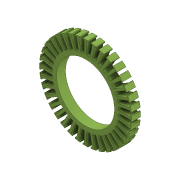
# Autodesk Inventor part: stator
Saved by Autodesk Inventor 2020 (Build 240168000, 168)
## iProperties
Created: 2020-05-19
Part Number: stator
Material: Generic
Document SubType Name: Modeling
Designer: Kostic
Density: 1 g/cm^3
Appearance: Olive Green
Author: Kostic
Autodesk Inventor part; units mm, degrees
ref_plane "YZ Plane" through (0, 0, 0) normal (1, 0, 0) x (0, 1, 0)
ref_plane "XZ Plane" through (0, 0, 0) normal (0, 1, 0) x (-1, 0, 0)
ref_plane "XY Plane" through (0, 0, 0) normal (0, 0, 1) x (1, 0, 0)
sketch "Sketch1" plane through (0, 0, 0) normal (0, 0, 1) x (1, 0, 0)
  circle A0 centre (0, 0) radius 26
  circle A1 centre (0, 0) radius 30
  line L0 (-1.1, 29.9798) -> (1.1, 29.9798)
  line L1 (1.1, 29.9798) -> (1.1, 41.4854)
  line L2 (1.1, 41.4854) -> (-1.1, 41.4854)
  line L3 (-1.1, 41.4854) -> (-1.1, 29.9798)
  circle A2 centre (0, 0) radius 41.5
  circle A3 centre (0, 0) radius 40.5
  line L4 (-2.3, 41.9535) -> (-2.3, 39.2792)
  line L5 (2.3, 41.9535) -> (2.3, 39.2792)
  point P0 (-1.1, 40.4851)
  point P1 (1.1, 40.4851)
  point P2 (2.3, 40.4346)
  point P3 (2.3, 41.4362)
  point P4 (-2.3, 41.4362)
  point P5 (-2.3, 40.4346)
  dimension "d1" = 60
  dimension "d2" = 83
  dimension "d0" = 52
  dimension "d3" = 81
  dimension "d4" = 1.1
  dimension "d5" = 2.2
  dimension "d7" = 2.3
  dimension "d8" = 2.3
  constraints: 12 end point, 4 coincident, 2 centre point, 2 parallel, 2 vertical, 1 horizontal, 1 perpendicular, 6 other
  measures "d0" diameter of A0
  measures "d3" diameter of A3
  measures "d4" distance from line of point (0, 0) L3
  measures "d5" distance between parallel lines of L1 L3
  measures "d7" distance from line of point (0, 0) L5
  measures "d8" distance from line of point (0, 0) L4
extrude "Extrusion1" add sketch "Sketch1" along normal blind 8 contours A1 L0 | A1 L3 A3 L1 | A3 L3 L2 L1 | L1 A2 L5 A3 | A3 L4 A2 L3 | L2 A2 picked at (28.1136, -4.5102) picked at (-0.8556, 33.4875)
pattern_circular "Circular Pattern1" count 36 over 360 about axis through (0, 0, 0) along (0, 0, 1) of "Extrusion1"
equation "\"d4\" = 0.5 * d5"
equation "\"d7\" = d8"
body "Solid1"
